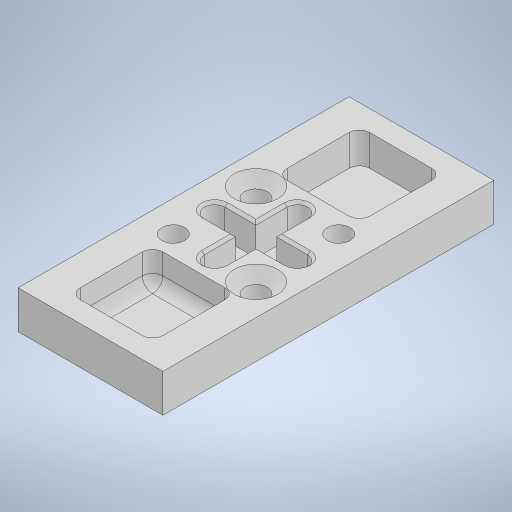
# Autodesk Inventor part: Recipe Test A
Saved by Autodesk Inventor 2023.2 (Build 272271000, 271)
## iProperties
Created: 2024-03-26
Part Number: Recipe Test A
Material: Generic
Document SubType Name: Modeling
Designer: Nathan Cai
Density: 1 g/cm^3
Appearance: Default
Author: Nathan Cai
Autodesk Inventor part; units mm, degrees
ref_plane "YZ Plane" through (0, 0, 0) normal (1, 0, 0) x (0, 1, 0)
ref_plane "XZ Plane" through (0, 0, 0) normal (0, 1, 0) x (-1, 0, 0)
ref_plane "XY Plane" through (0, 0, 0) normal (0, 0, 1) x (1, 0, 0)
sketch "Sketch1" plane through (0, 0, 0) normal (0, 1, 0) x (-1, 0, 0)
  line L0 (-11.1125, 25.4) -> (11.1125, 25.4)
  line L1 (11.1125, 25.4) -> (11.1125, -25.4)
  line L2 (11.1125, -25.4) -> (-11.1125, -25.4)
  line L3 (-11.1125, -25.4) -> (-11.1125, 25.4)
  line L4 (-11.1125, 25.4) -> (11.1125, -25.4) construction
  line L5 (11.1125, 25.4) -> (-11.1125, -25.4) construction
  point P0 (0, 0)
  dimension "d0" = 22.225
  dimension "d1" = 50.8
  constraints: 12 end point, 2 midpoint, 2 parallel, 1 horizontal, 1 perpendicular
  measures "d0" distance of L1.end L2.end
  measures "d1" distance of L0.end L1.end
extrude "Extrusion1" add sketch "Sketch1" along normal blind 5.842
sketch "Sketch2" plane through (0, 5.842, 0) normal (0, 1, 0) x (1, 0, 0)
  line L0 (-11.1125, -25.4) -> (11.1125, -25.4) construction
  line L1 (0, -25.4) -> (0, 25.4) construction
  line L2 (11.1125, 25.4) -> (-11.1125, 25.4) construction
  line L3 (-11.1125, 25.4) -> (-11.1125, -25.4) construction
  line L4 (-11.1125, 0) -> (11.1125, 0) construction
  line L5 (11.1125, -25.4) -> (11.1125, 25.4) construction
  line L6 (6.35, 0) -> (-6.35, 0) construction
  line L7 (6.35, 1.5875) -> (-6.35, 1.5875)
  line L8 (-6.35, -1.5875) -> (6.35, -1.5875)
  arc A0 (6.35, -1.5875) -> (6.35, 1.5875) centre (6.35, 0) ccw
  arc A1 (-6.35, 1.5875) -> (-6.35, -1.5875) centre (-6.35, 0) ccw
  line L9 (0, -6.35) -> (0, 6.35) construction
  line L10 (1.5875, -6.35) -> (1.5875, 6.35)
  line L11 (-1.5875, 6.35) -> (-1.5875, -6.35)
  arc A2 (-1.5875, -6.35) -> (1.5875, -6.35) centre (0, -6.35) ccw
  arc A3 (1.5875, 6.35) -> (-1.5875, 6.35) centre (0, 6.35) ccw
  line L12 (6.35, -22.225) -> (-6.35, -22.225)
  line L13 (-6.35, -22.225) -> (-6.35, -9.525)
  line L14 (-6.35, -9.525) -> (6.35, -9.525)
  line L15 (6.35, -9.525) -> (6.35, -22.225)
  line L16 (6.35, -22.225) -> (-6.35, -9.525) construction
  line L17 (-6.35, -22.225) -> (6.35, -9.525) construction
  line L18 (6.35, 22.225) -> (-6.35, 22.225)
  line L19 (-6.35, 22.225) -> (-6.35, 9.525)
  line L20 (-6.35, 9.525) -> (6.35, 9.525)
  line L21 (6.35, 9.525) -> (6.35, 22.225)
  line L22 (6.35, 22.225) -> (-6.35, 9.525) construction
  line L23 (-6.35, 22.225) -> (6.35, 9.525) construction
  line L24 (6.35, -6.35) -> (-6.35, -6.35) construction
  line L25 (-6.35, -6.35) -> (-6.35, 6.35) construction
  line L26 (-6.35, 6.35) -> (6.35, 6.35) construction
  line L27 (6.35, 6.35) -> (6.35, -6.35) construction
  line L28 (6.35, -6.35) -> (-6.35, 6.35) construction
  line L29 (-6.35, -6.35) -> (6.35, 6.35) construction
  circle A4 centre (-6.35, -6.35) radius 1.7526
  circle A5 centre (-6.35, 6.35) radius 1.7526
  circle A6 centre (6.35, -6.35) radius 1.7526
  circle A7 centre (6.35, 6.35) radius 1.7526
  point P0 (0, 0)
  point P1 (0, -15.875)
  point P2 (0, 15.875)
  point P3 (-1.5875, 1.5875)
  point P4 (-1.5875, -1.5875)
  point P5 (1.5875, -1.5875)
  point P6 (1.5875, 1.5875)
  dimension "d4" = 6.35
  dimension "d5" = 3.175
  dimension "d6" = 6.35
  dimension "d7" = 3.175
  dimension "d8" = 12.7
  dimension "d9" = 12.7
  dimension "d10" = 9.525
  dimension "d11" = 12.7
  dimension "d12" = 12.7
  dimension "d13" = 3.5052
  dimension "d14" = 3.5052
  dimension "d15" = 3.5052
  dimension "d16" = 3.5052
  constraints: 56 end point, 10 midpoint, 8 centre point, 8 point on circle, 8 tangent, 6 parallel, 5 symmetric about line, 4 coincident, 3 point on line, 2 horizontal, 2 perpendicular
  measures "d4" distance of point (0, 0) L6.end
  measures "d5" diameter of A1
  measures "d6" distance of point (0, 0) L9.end
  measures "d7" diameter of A3
  measures "d8" distance of L13.end L14.end
  measures "d9" distance of L12.end L13.end
  measures "d10" distance from line of L0 point (0, -15.875)
  measures "d11" distance of L25.end L26.end
  measures "d12" distance of L24.end L25.end
  measures "d13" diameter of A4
  measures "d14" diameter of A5
  measures "d15" diameter of A6
  measures "d16" diameter of A7
extrude "Extrusion2" cut sketch "Sketch2" against normal blind 4.7625
fillet "Fillet1" radius 1.5875 8 edges at (-6.35, 3.4608, 22.225) (-6.35, 3.4608, 9.525) (6.35, 3.4608, 22.225) (6.35, 3.4608, 9.525) (-6.35, 3.4608, -9.525) (-6.35, 3.4608, -22.225) (6.35, 3.4608, -22.225) (6.35, 3.4608, -9.525)
chamfer "Chamfer1" distance 1.5875 angle 45 2 edges at (4.5974, 5.842, 6.35) (-8.1026, 5.842, -6.35)
chamfer "Chamfer2" distance 0.3969 angle 45 12 edges at (-1.5875, 5.842, -3.9687) (0, 5.842, -7.9375) (1.5875, 5.842, -3.9687) (-3.9688, 5.842, -1.5875) (-7.9375, 5.842, 0) (-3.9687, 5.842, 1.5875) (-1.5875, 5.842, 3.9687) (0, 5.842, 7.9375) (1.5875, 5.842, 3.9687) (3.9687, 5.842, -1.5875) (7.9375, 5.842, 0) (3.9688, 5.842, 1.5875)
fillet "Fillet2" radius 1.5875 8 edges at (-5.885, 1.0795, 21.76) (-6.35, 1.0795, 15.875) (-5.885, 1.0795, 9.99) (0, 1.0795, 9.525) (5.885, 1.0795, 9.99) (6.35, 1.0795, 15.875) (5.885, 1.0795, 21.76) (0, 1.0795, 22.225)
body "Solid1"
